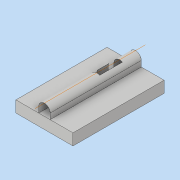
# Autodesk Inventor part: lw_5_корпус_new
Saved by Autodesk Inventor 2019 (Build 230136000, 136)
## iProperties
Created: 2021-04-29
Part Number: lw_5_корпус_new
Material: Типовые
Document SubType Name: Modeling
Designer: Kurbatova
Density: 1 g/cm^3
Appearance: По умолчанию
Author: Kurbatova
Autodesk Inventor part; units mm, degrees
ref_plane "YZ Plane" through (0, 0, 0) normal (1, 0, 0) x (0, 1, 0)
ref_plane "XZ Plane" through (0, 0, 0) normal (0, 1, 0) x (-1, 0, 0)
ref_plane "XY Plane" through (0, 0, 0) normal (0, 0, 1) x (1, 0, 0)
sketch "эскиз_корпус" plane through (0, 0, 0) normal (0, 0, 1) x (1, 0, 0)
  line L0 (0.9426, 4.9612) -> (-0.95, -5)
  line L1 (-5.05, 0) -> (5.05, 0)
  arc A0 (5.05, 0) -> (-5.05, 0) centre (0, 0) ccw
  line L2 (-5.05, 0) -> (-5.05, -5)
  line L3 (5.05, 0) -> (5.05, -5)
  arc A1 (5, 0) -> (-5, 0) centre (0, 0) ccw
  line L4 (-5.05, -5) -> (-5, -5)
  line L5 (5, -5) -> (5.05, -5)
  line L6 (5.05, -5) -> (25.05, -5)
  line L7 (-25.05, -5) -> (-5.05, -5)
  line L8 (-0.95, -5) -> (5, -5)
  line L9 (-0.95, -5) -> (-5, -5)
  line L10 (5, -5) -> (5, 0)
  line L11 (-5, 0) -> (-5, -5)
  line L12 (25.05, -5) -> (25.05, -15)
  line L13 (25.05, -15) -> (-25.05, -15)
  line L14 (-25.05, -15) -> (-25.05, -5)
  dimension "d33" = 5
  dimension "d34" = 5
  dimension "d52" = 0.05
  dimension "d85" = 10
  dimension "d89" = 20
  dimension "d91" = 20
  constraints: 30 end point, 5 horizontal, 5 point on circle, 3 perpendicular, 3 vertical, 2 centre point, 2 tangent, 1 coincident, 1 collinear, 1 midpoint, 1 point on line
  measures "d33" distance of L1.start L2.end
  measures "d34" distance of L1.end L3.end
  measures "d52" radial gap between concentric circles of A0 A1
  measures "d85" diameter of A1
  measures "d89" distance of L3.end L6.end
  measures "d91" distance of L7.start L2.end
extrude "корпус_общий" add sketch "эскиз_корпус" along normal blind 80
sketch "эскиз_отверстие_ручка" plane through (-5.05, -5, 0) normal (-1, 0, 0) x (0, 0, 1)
  line L0 (0, 0) -> (80, 0) projected
  line L1 (0, 5) -> (80, 5) projected
  line L2 (13.9957, 20) -> (13.9957, 0)
  line L3 (0, 0) -> (80, 0) projected
  line L4 (13.9957, 20) -> (33.9957, 20)
  line L5 (33.9957, 20) -> (33.9957, 0)
  line L6 (28.9957, 0) -> (28.9957, 7.5)
  line L7 (28.9957, 7.5) -> (18.9957, 7.5)
  line L8 (18.9957, 7.5) -> (18.9957, 0)
  line L9 (0, 5) -> (0, 5) projected
  line L10 (0, 5) -> (80, 5) projected
  line L11 (80, 5) -> (80, 5) projected
  line L12 (0, 5) -> (80, 5) projected
  line L13 (0, 10.05) -> (80, 10.05) projected
  line L14 (0, 5) -> (0, 10.05) projected
  line L15 (80, 5) -> (80, 10.05) projected
  dimension "d77" = 5
  dimension "d78" = 5
  dimension "d79" = 10
  dimension "d87" = 12.5
  dimension "d92" = 20
  constraints: 12 end point, 5 perpendicular, 4 point on line
  measures "d77" distance between parallel lines of L8 L2
  measures "d78" distance between parallel lines of L5 L6
  measures "d79" distance between parallel lines of L6 L8
  measures "d87" distance between parallel lines of L7 L4
  measures "d92" distance of L4.end L5.end
extrude "отверстие_ручка" cut sketch "эскиз_отверстие_ручка" against normal blind 7.5 contours L2 L1 L8 L0 | L2 L13 L5 L1 L6 L7 L8 | L6 L1 L5 L0 | L2 L4 L5 L13
extrude "отверстие_цилиндр" cut sketch "эскиз_корпус" along normal blind 80 contours A1 L1 L0 | L0 L1 A1 | L1 L10 L8 L0 | L0 L9 L11 L1
equation "\"d33\" = diametr_ruchka_"
equation "\"d34\" = diametr_ruchka_"
equation "\"d85\" = diametr_"
equation "\"d89\" = 2 * diametr_"
equation "\"d91\" = 2 * diametr_"
equation "\"d74\" = length"
equation "\"d77\" = diametr_ruchka_"
equation "\"d78\" = diametr_ruchka_"
equation "\"d79\" = diametr_"
equation "\"d87\" = 2.5 * diametr_ruchka_"
equation "\"d92\" = 2 * diametr_"
equation "\"d81\" = 1.5 * diametr_ruchka_"
equation "\"d83\" = length"
equation "\"diametr_ruchka_\" = 5"
equation "\"diametr_\" = 10"
equation "\"length\" = 80"
